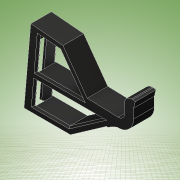
# Autodesk Inventor part: wall_hook
Saved by Autodesk Inventor 2017 (Build 210142000, 142)
## iProperties
Created: 2018-06-04
Part Number: wall_hook
Material: Generic
Document SubType Name: Modeling
Designer: Spark Electronics
Density: 1 g/cm^3
Appearance: Glossy - Black
Author: Spark Electronics
Autodesk Inventor part; units mm, degrees
ref_plane "YZ Plane" through (0, 0, 0) normal (1, 0, 0) x (0, 1, 0)
ref_plane "XZ Plane" through (0, 0, 0) normal (0, 1, 0) x (-1, 0, 0)
ref_plane "XY Plane" through (0, 0, 0) normal (0, 0, 1) x (1, 0, 0)
sketch "Sketch1" plane through (0, 0, 0) normal (0, 0, 1) x (1, 0, 0)
  line L0 (15.5971, 0.3833) -> (15.5971, -6.5123)
  line L1 (10.8185, -11.1464) -> (-12.0308, -10.4443)
  line L2 (0, -15.049) -> (0, 10.4443)
  arc A0 (10.8185, -11.1464) -> (15.5971, -6.5123) centre (10.9608, -6.5123) ccw
  line L3 (20.6771, 5.4633) -> (21.5633, 5.4633)
  line L4 (15.5971, -4.6694) -> (15.5971, 0.3833)
  arc A1 (20.6771, 5.4633) -> (15.5971, 0.3833) centre (20.6771, 0.3833) ccw
  line L5 (26.4264, -0.0507) -> (26.4501, 0)
  arc A2 (23.4995, 5.0798) -> (21.5633, 5.4633) centre (21.5633, 0.3833) ccw
  line L6 (3.4957, -21.3029) -> (2.1845, -21.3029)
  arc A3 (10.3183, -17.8224) -> (22.2892, -6.5123) centre (10.9608, -6.5123) ccw
  line L7 (22.2892, -6.5123) -> (22.2892, 0.3833)
  line L8 (22.2892, 0.3833) -> (23.4995, 5.0798)
  arc A4 (10.3183, -17.8224) -> (3.4957, -21.3029) centre (15.4342, -36.2781) ccw
  line L9 (-53.6218, 16.4218) -> (-56.9551, -21.6782)
  line L10 (-58.5479, -39.8843) -> (-56.9551, -21.6782)
  line L11 (-24.3241, -39.8843) -> (2.1845, -21.3029)
  line L12 (-24.3241, -39.8843) -> (-58.5479, -39.8843)
  line L13 (-12.0308, -10.4443) -> (-29.8499, 14.342)
  line L14 (-29.8499, 14.342) -> (-53.6218, 16.4218)
  line L15 (-51.7848, -35.4393) -> (-50.3031, -18.5036)
  line L16 (-50.3031, -18.5036) -> (-1.5661, -18.5036)
  line L17 (-1.5661, -18.5036) -> (-25.7269, -35.4393)
  line L18 (-25.7269, -35.4393) -> (-51.7848, -35.4393)
  line L19 (-49.8026, -12.7823) -> (-47.6834, 11.4402)
  line L20 (-47.6834, 11.4402) -> (-32.2687, 10.0916)
  line L21 (-32.2687, 10.0916) -> (-15.8244, -12.7823)
  line L22 (-15.8244, -12.7823) -> (-49.8026, -12.7823)
  point P0 (0, 0)
  dimension "d3" = 5.08
  dimension "d6" = 5
  dimension "d36" = 22.86
  dimension "d37" = 38.1
  dimension "d39" = 60.452
  dimension "d40" = 19.1516
  dimension "d41" = 11.3284
  dimension "d42" = 6.8955
  dimension "d43" = 4.6966
  dimension "d44" = 6.8955
  dimension "d45" = 4.6363
  dimension "d46" = 5.08
  dimension "d47" = 180
  dimension "d55" = 4.445
  dimension "d56" = 4.445
  dimension "d57" = 4.445
  dimension "d58" = 4.445
  dimension "d59" = 6.35
  dimension "d60" = 6.35
  constraints: 46 end point, 10 point on circle, 7 parallel, 5 centre point, 5 tangent, 4 horizontal, 1 perpendicular, 1 point on line, 1 vertical, 1 other
  measures "d3" radius of A1
  measures "d6" angle of L2 L9
  measures "d36" distance of L1.start L1.end
  measures "d37" vertical distance of L9.start L9.end
  measures "d39" distance of L6.start L9.end
  measures "d40" radius of A4
  measures "d41" radius of A3
  measures "d42" distance of L7.start L7.end
  measures "d43" vertical distance of L7.end L8.end
  measures "d44" distance of L0.start L0.end
  measures "d45" radius of A0
  measures "d46" radius of A2
  measures "d47" angle of L9 L10
  measures "d55" distance between parallel lines of L13 L21
  measures "d56" distance between parallel lines of L11 L17
  measures "d57" distance between parallel lines of L14 L20
  measures "d58" distance between parallel lines of L12 L18
  measures "d59" distance between parallel lines of L9 L19
  measures "d60" distance between parallel lines of L10 L15
extrude "Extrusion1" add sketch "Sketch1" along normal blind 15.24
ref_plane "Work Plane1" through (2.1845, -21.3029, 0) normal (-0.0871557, -0.9961947, 0) x (0, 0, 1)
sketch "Sketch2" plane through (2.1845, -21.3029, 0) normal (-0.0871557, -0.9961947, 0) x (0, 0, 1)
  line L0 (13.97, 51.7629) -> (11.4053, 57.2629)
  line L1 (1.27, 51.7629) -> (3.8347, 57.2629)
  line L2 (1.27, 51.7629) -> (13.97, 51.7629)
  line L3 (11.4053, 59.2629) -> (3.8347, 59.2629)
  line L4 (3.8347, 57.2629) -> (3.8347, 59.2629)
  line L5 (11.4053, 57.2629) -> (11.4053, 59.2629)
  line L6 (4.0347, 59.0629) -> (11.2053, 59.0629)
  line L7 (11.2053, 59.0629) -> (11.2053, 57.2185)
  line L8 (11.2053, 57.2185) -> (13.6561, 51.9629)
  line L9 (13.6561, 51.9629) -> (1.5839, 51.9629)
  line L10 (1.5839, 51.9629) -> (4.0347, 57.2185)
  line L11 (4.0347, 57.2185) -> (4.0347, 59.0629)
  line L12 (7.62, 58.7691) -> (7.62, 46.7298) construction
  line L13 (0, 58.8819) -> (15.24, 58.8819) projected
  line L14 (0, 58.8819) -> (0, 35.0191) projected
  point P0 (2.5708, 55.9125)
  point P1 (2.5708, 55.9125)
  dimension "d27" = 12.7
  dimension "d28" = 5.5
  dimension "d29" = 5.5
  dimension "d30" = 2
  dimension "d31" = 2
  dimension "d32" = 0.2
  dimension "d33" = 155
  dimension "d34" = 155
  dimension "d51" = 6.35
  dimension "d54" = 0.381
  dimension "d67" = 7.62
  constraints: 26 end point, 2 parallel, 2 perpendicular, 1 horizontal, 1 vertical, 5 other
  measures "d27" distance of L1.start L0.start
  measures "d28" distance from line of L2 L4.start
  measures "d29" distance from line of L2 L5.start
  measures "d30" distance of L4.start L4.end
  measures "d31" distance of L5.start L5.end
  measures "d32" distance between parallel lines of L4 L11
  measures "d33" angle of L1 L4
  measures "d34" angle of L0 L5
  measures "d51" distance from line of L1.start L12
  measures "d54" distance between parallel lines of L13 L3
  measures "d67" distance between parallel lines of L12 L14
extrude "Extrusion2" cut sketch "Sketch2" along normal blind 25.4 and the other way blind 25.4
chamfer "Chamfer3" distance 1.27 angle 45 16 edges at (-24.0466, -1.3453, 15.24) (-24.0466, -1.3453, 0) (-13.6465, -26.9715, 15.24) (-13.6465, -26.9715, 0) (-48.743, -0.671, 15.24) (-48.743, -0.671, 0) (-51.0439, -26.9715, 15.24) (-51.0439, -26.9715, 0) (-32.8135, -12.7823, 15.24) (-32.8135, -12.7823, 0) (-38.7558, -35.4393, 15.24) (-38.7558, -35.4393, 0) (-25.9346, -18.5036, 15.24) (-25.9346, -18.5036, 0) (-39.976, 10.7659, 15.24) (-39.976, 10.7659, 0)
body "Solid1"
